# Autodesk Inventor part: bottomPlate
Saved by Autodesk Inventor 2015 SP1 (Build 190203100, 203)
## iProperties
Created: 2015-02-12
Part Number: bottomPlate
Material: Generic
Document SubType Name: Modeling
Designer: Jostein
Density: 1 g/cm^3
Appearance: Default
Author: Jostein
Autodesk Inventor part; units mm, degrees
ref_plane "YZ Plane" through (0, 0, 0) normal (1, 0, 0) x (0, 1, 0)
ref_plane "XZ Plane" through (0, 0, 0) normal (0, 1, 0) x (-1, 0, 0)
ref_plane "XY Plane" through (0, 0, 0) normal (0, 0, 1) x (1, 0, 0)
sketch "Sketch1" plane through (0, 0, 0) normal (0, 0, 1) x (1, 0, 0)
  circle A0 centre (0, 0) radius 245
  dimension "d0" = 490
  constraints: 1 centre point, 1 coincident
  measures "d0" diameter of A0
extrude "Extrusion1" add sketch "Sketch1" along normal blind 3
sketch "Sketch2" plane through (0, 0, 3) normal (0, 0, 1) x (1, 0, 0)
  line L0 (0, 0) -> (154, 0) construction
  circle A0 centre (154, 0) radius 12
  circle A1 centre (-77, 133.3679) radius 12
  circle A2 centre (-77, -133.3679) radius 12
  dimension "d3" = 154
  dimension "d4" = 24
  dimension "d7" = 360
  constraints: 3 centre point, 2 end point, 1 coincident, 1 horizontal alignment, 7 other
  measures "d3" distance of L0.start L0.end
  measures "d4" diameter of A0
extrude "Extrusion2" cut sketch "Sketch2" against normal through all
body "Solid1"
